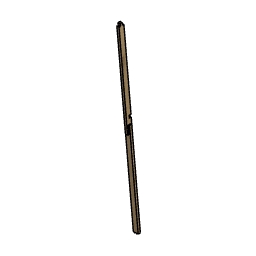
pedalboard1_piedcoupe v7 (Autodesk Fusion 360 archive; units mm, degrees)
design "piedcourt"
Autodesk Fusion 360 part; units mm, degrees
note: some values were not read from the file. Chosen so that the rebuilt part matches the saved one: which face or edge a step refers to. Set by a fixed rule: which sketch regions a step uses.
imported_body "Fonction de base1" makes body 1
move_body "Desplazar1" bodies 1 to x (1, 0, 0) y (0, 1, 0) z (0, 0, 1) at (10, -40, 100)
move_body "Desplazar2" bodies 1 to x (1, 0, 0) y (0, 1, 0) z (0, 0, 1) at (0, 0, -0.4)
move_body "Desplazar3" bodies 1 to x (1, 0, 0) y (0, 1, 0) z (0, 0, 1) at (0, 0, -13)
copy_body "CopiarPegarCuerpos1" bodies 1 makes body 2
move_body "Desplazar4" bodies 2 to x (1, 0, 0) y (0, 1, 0) z (0, 0, 1) at (0, -40, 450)
move_body "Alinear2" bodies 2 to x (1, 0, 0) y (0, 1, 0) z (0, 0, 1) at (0, 0.6253, 0.0547)
sketch "Boceto3" plane through (210, 0, 0) normal (1, 0, 0) x (0, 1, 0)
  line L0 (123.108, -860.8821) -> (114.2331, -860.8821)
  line L1 (114.2331, -860.8821) -> (114.2331, -850.8821)
  line L2 (114.2331, -850.8821) -> (122.2331, -850.8821)
  line L3 (122.2331, -850.8821) -> (50.3827, -29.6284)
  line L4 (50.3827, -29.6284) -> (44.3827, -29.6284)
  line L5 (44.3827, -29.6284) -> (43.5111, -19.6664)
  line L6 (43.5111, -19.6664) -> (33.5111, -19.6664)
  line L7 (33.5111, -19.6664) -> (34.3827, -29.6284)
  line L8 (34.3827, -29.6284) -> (28.3827, -29.6284)
  line L9 (28.3827, -29.6284) -> (106.8229, -926.2036)
  line L10 (106.8229, -926.2036) -> (128.8229, -926.2036)
  line L11 (128.8229, -926.2036) -> (123.108, -860.8821)
  line L12 (83.7333, -410.8274) -> (74.8584, -410.8274)
  line L13 (74.8584, -410.8274) -> (74.8584, -400.8274)
  line L14 (74.8584, -400.8274) -> (82.8584, -400.8274)
  line L15 (82.8584, -400.8274) -> (11.008, 420.4263)
  line L16 (11.008, 420.4263) -> (5.008, 420.4263)
  line L17 (5.008, 420.4263) -> (4.1364, 430.3883)
  line L18 (4.1364, 430.3883) -> (-5.8636, 430.3883)
  line L19 (-5.8636, 430.3883) -> (-4.992, 420.4263)
  line L20 (-4.992, 420.4263) -> (-10.992, 420.4263)
  line L21 (-10.992, 420.4263) -> (67.4482, -476.1489)
  line L22 (67.4482, -476.1489) -> (89.4482, -476.1489)
  line L23 (89.4482, -476.1489) -> (83.7333, -410.8274)
  line L24 (28.3827, -29.6284) -> (34.3827, -29.6284)
  line L25 (33.5111, -19.6664) -> (43.5111, -19.6664)
  line L26 (33.5111, -19.6664) -> (34.3827, -29.6284)
  line L27 (43.5111, -19.6664) -> (44.3827, -29.6284)
  line L28 (44.3827, -29.6284) -> (50.3827, -29.6284)
  line L29 (50.3827, -29.6284) -> (82.8584, -400.8274)
  line L30 (82.8584, -400.8274) -> (74.8584, -400.8274)
  line L31 (74.8584, -400.8274) -> (74.8584, -410.8274)
  line L32 (74.8584, -410.8274) -> (83.7333, -410.8274)
  line L33 (83.7333, -410.8274) -> (89.4482, -476.1489)
  line L34 (89.4482, -476.1489) -> (67.4482, -476.1489)
  line L35 (67.4482, -476.1489) -> (28.3827, -29.6284)
  line L36 (82.8584, -400.3274) -> (74.8584, -400.3274)
  line L37 (74.8584, -411.3274) -> (83.777, -411.3274)
  line L38 (82.8584, -400.3274) -> (82.8584, -400.8274)
  line L39 (82.8584, -400.8274) -> (74.8584, -400.8274)
  line L40 (74.8584, -400.8274) -> (74.8584, -400.3274)
  line L41 (74.8584, -400.3274) -> (82.8584, -400.3274)
  line L42 (82.8147, -400.3274) -> (82.8584, -400.3274)
  line L43 (74.8584, -410.8274) -> (74.8584, -411.3274)
  line L44 (74.8584, -411.3274) -> (83.777, -411.3274)
  line L45 (83.777, -411.3274) -> (83.7333, -410.8274)
  line L46 (83.7333, -410.8274) -> (74.8584, -410.8274)
  dimension "d15" = 0.5
  constraint coincident L8.end L9.start
  constraint coincident L7.end L8.start
  constraint coincident L6.end L7.start
  constraint coincident L5.end L6.start
  constraint coincident L4.end L5.start
  constraint coincident L3.end L4.start
  constraint coincident L14.end L15.start
  constraint coincident L13.end L14.start
  constraint coincident L12.end L13.start
  constraint coincident L12.start L23.end
  constraint coincident L22.end L23.start
  constraint coincident L21.end L22.start
  constraint perpendicular L30 L38
  constraint perpendicular L40 L41
  constraint coincident L41 L42.start
  constraint coincident L29 L42.start
  constraint perpendicular L37 L43
  constraint coincident L3 L37.end
extrude "Extruir1" add sketch "Boceto3" along normal blind 10 separate body contours L3 L4 L5 L6 L7 L8 L9 L13 L15 L21 L22 L23 L24 L25 L26 L27 L28 L29 L31 L33 L34 L35 L36 L37 L40 L41 L43 L44 makes body 3
sketch "Boceto5" plane through (220, 0, 0) normal (1, 0, 0) x (0, 1, 0)
  line L0 (33.5111, -19.6664) -> (34.3827, -29.6284)
  line L1 (34.3827, -29.6284) -> (28.3827, -29.6284)
  line L2 (28.3827, -29.6284) -> (67.4482, -476.1489)
  line L3 (67.4482, -476.1489) -> (89.4482, -476.1489)
  line L4 (89.4482, -476.1489) -> (83.777, -411.3274)
  line L5 (74.8584, -411.3274) -> (74.8584, -400.3274)
  line L6 (82.8147, -400.3274) -> (50.3827, -29.6284)
  line L7 (50.3827, -29.6284) -> (44.3827, -29.6284)
  line L8 (44.3827, -29.6284) -> (43.5111, -19.6664)
  line L9 (43.5111, -19.6664) -> (33.5111, -19.6664)
  circle A0 centre (32.8268, -29.6284) radius 1.55
  circle A1 centre (45.9386, -29.6284) radius 1.55
  circle A2 centre (74.8584, -401.8774) radius 1.55
  circle A3 centre (74.8584, -409.7774) radius 1.55
  line L10 (74.8584, -400.3274) -> (82.8147, -400.3274)
  line L11 (83.777, -411.3274) -> (74.8584, -411.3274)
  dimension "d9" = 3.1
  dimension "d10" = 3.1
  dimension "d11" = 3.1
  dimension "d12" = 3.1
  constraint coincident L1 A0.centre
  constraint coincident L7 A1.centre
  constraint tangent L0 A0
  constraint tangent L8 A1
  constraint coincident L5 A2.centre
  constraint coincident L5 A3.centre
  constraint tangent A2 L10
  constraint tangent A3 L11
  measures "d9" diameter of A0
  measures "d10" diameter of A1
  measures "d11" diameter of A2
  measures "d12" diameter of A3
extrude "Extruir3" cut sketch "Boceto5" against normal blind 13 contours L1 A0 | L7 A1 | L5 A3 | L5 A3 | L5 A2 | L5 A2 picked at (33.3434, -30.2105) picked at (45.6107, -30.1093) bodies 3
sketch "Esquisse6" plane through (220, 0, 0) normal (1, 0, 0) x (0, 1, 0)
  arc A0 (74.8584, -408.2274) -> (74.8584, -411.3274) centre (74.8584, -409.7774) ccw
  line L0 (74.8584, -408.2274) -> (74.8584, -403.4274)
  arc A1 (74.8584, -400.3274) -> (74.8584, -403.4274) centre (74.8584, -401.8774) ccw
  line L1 (74.8584, -400.3274) -> (82.8147, -400.3274)
  line L2 (82.8147, -400.3274) -> (50.3827, -29.6284)
  line L3 (50.3827, -29.6284) -> (47.4886, -29.6284)
  arc A2 (44.3886, -29.6284) -> (47.4886, -29.6284) centre (45.9386, -29.6284) ccw
  line L4 (44.3886, -29.6284) -> (44.3827, -29.6284)
  line L5 (44.3827, -29.6284) -> (43.5111, -19.6664)
  line L6 (43.5111, -19.6664) -> (33.5111, -19.6664)
  line L7 (33.5111, -19.6664) -> (34.3827, -29.6284)
  line L8 (34.3827, -29.6284) -> (34.3768, -29.6284)
  arc A3 (31.2768, -29.6284) -> (34.3768, -29.6284) centre (32.8268, -29.6284) ccw
  line L9 (31.2768, -29.6284) -> (28.3827, -29.6284)
  line L10 (28.3827, -29.6284) -> (67.4482, -476.1489)
  line L11 (67.4482, -476.1489) -> (89.4482, -476.1489)
  line L12 (89.4482, -476.1489) -> (83.777, -411.3274)
  line L13 (83.777, -411.3274) -> (74.8584, -411.3274)
  line L14 (67.4482, -476.1489) -> (28.3827, -29.6284)
  line L15 (28.3827, -29.6284) -> (31.2768, -29.6284)
  arc A4 (31.2768, -29.6284) -> (34.3768, -29.6284) centre (32.8268, -29.6284) ccw
  line L16 (34.3768, -29.6284) -> (33.5111, -19.6664)
  line L17 (33.5111, -19.6664) -> (43.5111, -19.6664)
  line L18 (43.5111, -19.6664) -> (44.3827, -29.6284)
  arc A5 (44.3827, -29.6284) -> (47.4945, -29.6284) centre (45.9386, -29.6284) ccw
  line L19 (47.4945, -29.6284) -> (50.3827, -29.6284)
  line L20 (50.3827, -29.6284) -> (89.4482, -476.1489)
  line L21 (78.4482, -476.1489) -> (76.6601, -455.7114) construction
  line L22 (76.6601, -455.7114) -> (81.6601, -455.274) construction
  line L23 (81.6601, -455.274) -> (76.6601, -455.7114) construction
  line L24 (76.6601, -455.7114) -> (71.6601, -456.1489) construction
  line L25 (71.6601, -456.1489) -> (73.4099, -476.1489) construction
  line L26 (81.6601, -455.274) -> (83.4864, -476.1489) construction
  line L27 (73.4099, -476.1489) -> (71.6601, -456.1489)
  line L28 (71.6601, -456.1489) -> (81.6601, -455.274)
  line L29 (81.6601, -455.274) -> (83.4864, -476.1489)
  line L30 (83.4864, -476.1489) -> (89.4482, -476.1489)
  line L31 (73.4099, -476.1489) -> (67.4482, -476.1489)
  dimension "d17" = 5
  dimension "d18" = 5
  dimension "d21" = 20
  constraint coincident L10.end L11.start
  constraint coincident L9.end L10.start
  constraint coincident A3.start L9.start
  constraint coincident A3.centre A4.centre
  constraint coincident L8.end A3.end
  constraint coincident L6.end L7.start
  constraint coincident L5.end L6.start
  constraint coincident L4.end L5.start
  constraint coincident A2.centre A5.centre
  constraint coincident L2.end L3.start
  constraint parallel L3 L19
  constraint coincident L11.end L12.start
  constraint midpoint L11 L21.start
  constraint parallel L12 L21
  constraint perpendicular L21 L22
  constraint perpendicular L21 L24
  constraint coincident L11 L25.end
  constraint perpendicular L24 L25
  constraint coincident L11 L26.end
  constraint perpendicular L23 L26
  measures "d17" horizontal distance of L21.end L24.end
  measures "d18" horizontal distance of L21.end L22.end
  measures "d21" vertical distance of L24.end L25.end
extrude "Extrusion4" add sketch "Esquisse6" along normal blind 10 separate body contours A0 L0 A1 L1 L2 L3 L5 L6 L7 L8 A3 L9 L10 L11 L12 L13 L14 L15 A4 L17 L18 A5 L19 L20 L27 L28 L29 L30 L31 makes body 4
sketch "Esquisse7" plane through (230, 0, 0) normal (1, 0, 0) x (0, 1, 0)
  line L0 (71.6601, -456.1489) -> (81.6601, -455.274)
  line L1 (81.6601, -455.274) -> (83.4864, -476.1489)
  line L2 (83.4864, -476.1489) -> (89.4482, -476.1489)
  line L3 (89.4482, -476.1489) -> (83.777, -411.3274)
  line L4 (50.3827, -29.6284) -> (47.4945, -29.6284)
  arc A0 (44.3827, -29.6284) -> (47.4945, -29.6284) centre (45.9386, -29.6284) ccw
  line L5 (44.3827, -29.6284) -> (43.5111, -19.6664)
  line L6 (43.5111, -19.6664) -> (33.5111, -19.6664)
  line L7 (33.5111, -19.6664) -> (34.3827, -29.6284)
  line L8 (34.3827, -29.6284) -> (34.3768, -29.6284)
  arc A1 (31.2768, -29.6284) -> (34.3768, -29.6284) centre (32.8268, -29.6284) ccw
  line L9 (31.2768, -29.6284) -> (28.3827, -29.6284)
  line L10 (28.3827, -29.6284) -> (67.4482, -476.1489)
  line L11 (67.4482, -476.1489) -> (73.4099, -476.1489)
  line L12 (73.4099, -476.1489) -> (71.6601, -456.1489)
  line L13 (67.4482, -476.1489) -> (73.4099, -476.1489)
  line L14 (73.4099, -476.1489) -> (71.6601, -456.1489)
  line L15 (71.6601, -456.1489) -> (81.6601, -455.274)
  line L16 (81.6601, -455.274) -> (83.4864, -476.1489)
  line L17 (83.4864, -476.1489) -> (89.4482, -476.1489)
  line L18 (89.4482, -476.1489) -> (83.777, -411.3274)
  line L19 (28.3827, -29.6284) -> (67.4482, -476.1489)
  line L20 (83.777, -411.3274) -> (74.8584, -411.3274)
  arc A2 (74.8584, -408.2274) -> (74.8584, -411.3274) centre (74.8584, -409.7774) ccw
  line L21 (74.8584, -408.2274) -> (74.8584, -403.4274)
  arc A3 (74.8584, -400.3274) -> (74.8584, -403.4274) centre (74.8584, -401.8774) ccw
  line L22 (74.8584, -400.3274) -> (82.8147, -400.3274)
  line L23 (82.8147, -400.3274) -> (50.3827, -29.6284)
  line L24 (83.777, -411.3274) -> (50.3827, -29.6284)
  line L25 (50.3827, -29.6284) -> (28.3827, -29.6284)
  constraint coincident L10.end L11.start
  constraint coincident L11.end L12.start
  constraint coincident L0.start L12.end
  constraint coincident L0.end L1.start
  constraint coincident L1.end L2.start
  constraint coincident L2.end L3.start
  constraint coincident L3.end L18.end
  constraint coincident L9.end L10.start
  constraint coincident L4.start L23.end
extrude "Extrusion5" add sketch "Esquisse7" along normal blind 10 separate body contours L0 L1 L2 L3 L4 A0 L8 A1 L9 L10 L11 L12 L13 L14 L15 L16 L17 L18 L19 L20 A2 L21 A3 L22 L23 L24 L25 | L20 A2 L21 A3 L22 L24 | A1 L25 | A0 L25 makes body 5
move_body "Déplacer5" bodies 5 to x (0, 0.996195, 0.087156) y (0.996195, -0.007596, 0.086824) z (0.087156, 0.086824, -0.992404) at (188.6728, -117.2162, -936.017)
move_body "Déplacer6" bodies 2 to x (0, 0.996195, 0.087156) y (0.996195, -0.007596, 0.086824) z (0.087156, 0.086824, -0.992404) at (187.6966, -58.8981, -1261.2141)
move_body "Aligner3" bodies 2 to x (1, 0, 0) y (0, 1, 0) z (0, 0, 1) at (0, 0.2456, 0.0215)
move_body "Aligner4" bodies 2 to x (1, 0, 0) y (0, 1, 0) z (0, 0, 1) at (0.9762, 0, 0)
sketch "Esquisse8" plane through (0, 31.5301, 2.7585) normal (0, -0.996195, -0.087156) x (1, 0, 0)
  line L0 (214.3652, -890.2498) -> (236.2815, -888.3324)
  line L1 (236.2815, -888.3324) -> (236.2815, -440.1062)
  line L2 (236.2815, -440.1062) -> (230.3424, -440.6258)
  line L3 (230.3424, -440.6258) -> (230.3424, -461.5804)
  line L4 (230.3424, -461.5804) -> (220.3042, -461.5804)
  line L5 (220.3042, -461.5804) -> (220.3042, -441.504)
  line L6 (220.3042, -441.504) -> (214.3652, -442.0236)
  line L7 (214.3652, -442.0236) -> (214.3652, -890.2498)
  line L8 (227.4404, -835.4931) -> (236.2815, -834.7196)
  line L9 (236.2815, -834.7196) -> (236.2815, -769.1486)
  line L10 (236.2815, -769.1486) -> (214.3652, -771.066)
  line L11 (214.3652, -771.066) -> (214.3652, -1671.066)
  line L12 (214.3652, -1671.066) -> (220.3424, -1670.5431)
  line L13 (220.3424, -1670.5431) -> (220.3424, -1680.5431)
  line L14 (220.3424, -1680.5431) -> (230.3043, -1679.6715)
  line L15 (230.3043, -1679.6715) -> (230.3043, -1669.6715)
  line L16 (230.3043, -1669.6715) -> (236.2815, -1669.1486)
  line L17 (236.2815, -1669.1486) -> (236.2815, -844.7578)
  line L18 (236.2815, -844.7578) -> (228.3119, -845.455)
  line L19 (228.3119, -845.455) -> (227.4404, -835.4931)
  line L20 (236.2815, -834.7196) -> (227.4404, -835.4931)
  line L21 (227.4404, -835.4931) -> (228.3119, -845.455)
  line L22 (228.3119, -845.455) -> (236.2815, -844.7578)
  line L23 (236.2815, -834.3181) -> (227.007, -835.1295)
  line L24 (227.007, -835.1295) -> (227.9483, -845.8884)
  line L25 (227.9483, -845.8884) -> (236.3163, -845.1563)
  circle A0 centre (227.1421, -836.6736) radius 1.55
  circle A1 centre (227.8132, -844.3443) radius 1.55
  dimension "d27" = 3.1
  dimension "d28" = 3.1
  constraint coincident L8.end L9.start
  constraint coincident L8.start L19.end
  constraint coincident L18.end L19.start
  constraint coincident L17.end L18.start
  constraint coincident L24 A0.centre
  constraint tangent L23 A0
  constraint coincident L24 A1.centre
  constraint tangent L25 A1
  constraint coincident L1 L23.start
  measures "d27" diameter of A0
  measures "d28" diameter of A1
extrude "Extrusion6" cut sketch "Esquisse8" against normal blind 15 contours L1 L17 L18 L22 L25 A1 | L1 L8 L18 L19 L20 L21 L22 A0 A1 | L24 A1 | L18 L19 L21 L22 L24 A1 | L1 L8 L9 L20 L23 A0 | L18 L19 L21 L22 A1 | L19 L21 L24 A0 A1 | L8 L19 L20 L21 L24 A0 | L24 A0 | L8 L19 L20 L21 A0 bodies 5
copy_body "Corps->Comp1" bodies 4 removing the originals makes body 6 in component "haut_pied"
copy_body "Corps->Comp2" bodies 5 removing the originals makes body 7 in component "bas_pied"
sketch "Esquisse9" plane through (0, 31.5301, 2.7585) normal (0, -0.996195, -0.087156) x (1, 0, 0)
  line L0 (227.007, -835.1295) -> (236.2815, -834.3181)
  line L1 (236.2815, -834.3181) -> (236.2815, -440.1062)
  line L2 (236.2815, -440.1062) -> (230.3424, -440.6258)
  line L3 (230.3424, -440.6258) -> (230.3424, -461.5804)
  line L4 (230.3424, -461.5804) -> (220.3042, -461.5804)
  line L5 (220.3042, -461.5804) -> (220.3042, -441.504)
  line L6 (220.3042, -441.504) -> (214.3652, -442.0236)
  line L7 (214.3652, -442.0236) -> (214.3652, -890.2498)
  line L8 (214.3652, -890.2498) -> (236.2815, -888.3324)
  line L9 (236.2815, -888.3324) -> (236.2815, -845.1593)
  line L10 (236.2815, -845.1593) -> (227.9483, -845.8884)
  arc A0 (227.6781, -842.8002) -> (227.9483, -845.8884) centre (227.8132, -844.3443) ccw
  line L11 (227.6781, -842.8002) -> (227.2772, -838.2177)
  arc A1 (227.007, -835.1295) -> (227.2772, -838.2177) centre (227.1421, -836.6736) ccw
  line L12 (236.2815, -845.1593) -> (227.9483, -845.8884)
  line L13 (236.2815, -834.3181) -> (227.007, -835.1295)
  arc A2 (227.007, -835.1295) -> (227.2772, -838.2177) centre (227.1421, -836.6736) ccw
  arc A3 (227.8132, -842.7943) -> (227.9483, -845.8884) centre (227.8132, -844.3443) ccw
  line L14 (227.6781, -842.8002) -> (227.2772, -838.2177)
  line L15 (236.2815, -834.3181) -> (236.2815, -845.1593)
  constraint coincident L9.end L10.start
  constraint coincident L10.end A0.end
  constraint coincident L0.end L1.start
  constraint coincident L0.start A1.start
  constraint coincident L11.end A1.end
  constraint coincident A1.centre A2.centre
  constraint coincident A0.centre A3.centre
  constraint coincident A0.start L11.start
extrude "Extrusion1" add sketch "Esquisse9" against normal blind 10 contours L0 L10 A0 L11 A1 L12 L13 A2 A3 L14 L15 bodies 7 in component "bas_pied"
component "haut_pied" placed x (1, 0, 0) y (0, 1, 0) z (0, 0, 1) at (0, 0, 0)
component "bas_pied" placed x (1, 0, 0) y (0, 1, 0) z (0, 0, 1) at (0, 0, 0)
hidden bodies 1 2 3
named bodies: "pie4", "pie4 (1)", "haut_pied", "bas_pied"
